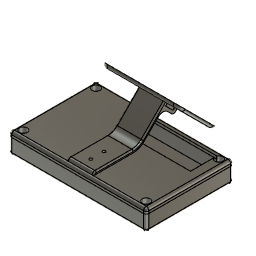
LCD 2004 (Autodesk Fusion 360 design; units mm, degrees)
Autodesk Fusion 360 part; units mm, degrees
sketch "base" plane through (0, 0, 0) normal (0, 0, 1) x (1, 0, 0)
  line L0 (0, 0) -> (104, 0)
  line L1 (104, 0) -> (104, 66)
  line L2 (104, 66) -> (0, 66)
  line L3 (0, 66) -> (0, 0)
  line L4 (2, 53) -> (102, 53)
  line L5 (102, 53) -> (102, 13)
  line L6 (102, 13) -> (2, 13)
  line L7 (2, 13) -> (2, 53)
  line L8 (2, 53) -> (102, 53)
  line L9 (102, 53) -> (102, 64)
  line L10 (102, 64) -> (2, 64)
  line L11 (2, 64) -> (2, 53)
  line L12 (2, 13) -> (102, 13)
  line L13 (102, 13) -> (102, 2)
  line L14 (102, 2) -> (2, 2)
  line L15 (2, 2) -> (2, 13)
  line L16 (2, 53) -> (3, 53)
  line L17 (3, 53) -> (3, 13)
  line L18 (3, 13) -> (2, 13)
  line L19 (2, 13) -> (2, 53)
  line L20 (102, 53) -> (101, 53)
  line L21 (101, 53) -> (101, 13)
  line L22 (101, 13) -> (102, 13)
  line L23 (102, 13) -> (102, 53)
  dimension "d1" = 104
  dimension "d2" = 66
  dimension "d3" = 100
  dimension "d4" = 40
  dimension "d6" = 2
  dimension "d8" = 11
  dimension "d10" = 11
  dimension "d41" = 2
  dimension "d46" = 1
  dimension "d47" = 1
  constraint horizontal L0
  constraint vertical L1
  constraint horizontal L2
  constraint vertical L3
  constraint coincident L0.start L3.end
  constraint horizontal L4
  constraint vertical L5
  constraint horizontal L6
  constraint vertical L7
  constraint horizontal L8
  constraint vertical L9
  constraint horizontal L10
  constraint vertical L11
  constraint horizontal L12
  constraint vertical L13
  constraint horizontal L14
  constraint vertical L15
  constraint coincident L5.end L13
  constraint coincident L4.end L9
  constraint horizontal L16
  constraint vertical L17
  constraint horizontal L18
  constraint vertical L19
  constraint horizontal L20
  constraint vertical L21
  constraint horizontal L22
  constraint vertical L23
  measures "d1" distance of L0.start L0.end
  measures "d2" distance of L0.start L2.end
  measures "d3" distance of L4.start L4.end
  measures "d4" distance of L4.start L6.end
  measures "d6" distance of L3 L7
  measures "d8" distance of L4.start L10.end
  measures "d10" distance of L6.end L14.end
  measures "d41" distance of L2 L10
  measures "d46" distance of L4.start L16.end
  measures "d47" distance of L4.end L20.end
extrude "Extrude1" add sketch "base" along normal blind 2 contours L4 L8 L9 L10 L11 L16 L20 | L4 L6 L7 L8 L12 L16 L17 L18 L19 | L6 L12 L13 L14 L15 L18 L22 | L4 L5 L6 L8 L12 L20 L21 L22 L23 makes body 1
extrude "Extrude2" add sketch "base" along normal blind 12 bodies 1
fillet "Fillet1" radius 2 4 edges at (0, 0, 6) (0, 66, 6) (104, 66, 6) (104, 0, 6) on bodies 1
fillet "Fillet2" radius 2 8 edges at (104, 33, 0) (103.4142, 65.4142, 0) (52, 66, 0) (0.5858, 65.4142, 0) (0, 33, 0) (0.5858, 0.5858, 0) (52, 0, 0) (103.4142, 0.5858, 0) on bodies 1
sketch "stands " plane through (0, 0, 2) normal (0, 0, 1) x (-1, 0, 0)
  line L0 (-2, -2) -> (-102, -2)
  line L1 (-102, -2) -> (-102, -64)
  line L2 (-101, -13) -> (-3, -13)
  line L3 (-2, -64) -> (-2, -2)
  line L4 (-2, -64) -> (-11, -64)
  line L5 (-11, -64) -> (-11, -55)
  line L6 (-11, -55) -> (-2, -55)
  line L7 (-2, -55) -> (-2, -64)
  line L8 (-102, -64) -> (-93, -64)
  line L9 (-93, -64) -> (-93, -55)
  line L10 (-93, -55) -> (-102, -55)
  line L11 (-102, -55) -> (-102, -64)
  line L12 (-102, -2) -> (-93, -2)
  line L13 (-93, -2) -> (-93, -11)
  line L14 (-93, -11) -> (-102, -11)
  line L15 (-102, -11) -> (-102, -2)
  line L16 (-2, -2) -> (-11, -2)
  line L17 (-11, -2) -> (-11, -11)
  line L18 (-11, -11) -> (-2, -11)
  line L19 (-2, -11) -> (-2, -2)
  circle A0 centre (-5.4, -60.6) radius 2.2
  circle A1 centre (-98.6, -60.6) radius 2.2
  circle A2 centre (-98.6, -5.4) radius 2.2
  circle A3 centre (-5.4, -5.4) radius 2.2
  line L20 (-3, -13) -> (-3, -53)
  line L21 (-3, -53) -> (-101, -53)
  line L22 (-101, -53) -> (-101, -13)
  line L23 (-102, -64) -> (-2, -64)
  point P0 (-2, -64)
  point P1 (-102, -64)
  dimension "d19" = 9
  dimension "d20" = 9
  dimension "d21" = 9
  dimension "d22" = 9
  dimension "d23" = 9
  dimension "d24" = 9
  dimension "d25" = 9
  dimension "d26" = 9
  dimension "d29" = 4.4
  dimension "d30" = 4.4
  dimension "d31" = 4.4
  dimension "d32" = 4.4
  dimension "d33" = 3.4
  dimension "d34" = 3.4
  dimension "d35" = 3.4
  dimension "d36" = 3.4
  dimension "d37" = 3.4
  dimension "d38" = 3.4
  dimension "d39" = 3.4
  dimension "d40" = 3.4
  constraint horizontal L4
  constraint vertical L5
  constraint horizontal L6
  constraint vertical L7
  constraint horizontal L8
  constraint vertical L9
  constraint horizontal L10
  constraint vertical L11
  constraint horizontal L12
  constraint vertical L13
  constraint horizontal L14
  constraint vertical L15
  constraint coincident L0.end L1.start
  constraint horizontal L16
  constraint vertical L17
  constraint horizontal L18
  constraint vertical L19
  constraint coincident L0.start L3.end
  constraint coincident L4 P0
  constraint coincident L7 P0
  constraint coincident L8 P1
  constraint coincident L11 P1
  measures "d19" distance of P0 L4.end
  measures "d20" distance of P0 L6.end
  measures "d21" distance of P1 L8.end
  measures "d22" distance of P1 L10.end
  measures "d23" distance of L0.end L12.end
  measures "d24" distance of L0.end L14.end
  measures "d25" distance of L0.start L16.end
  measures "d26" distance of L0.start L18.end
  measures "d29" diameter of A0
  measures "d30" diameter of A1
  measures "d31" diameter of A2
  measures "d32" diameter of A3
  measures "d33" distance of L19 A3.centre
  measures "d34" distance of L16 A3.centre
  measures "d35" distance of L15 A2.centre
  measures "d36" distance of L12 A2.centre
  measures "d37" distance of L11 A1.centre
  measures "d38" distance of L8 A1.centre
  measures "d39" distance of L7 A0.centre
  measures "d40" distance of L4 A0.centre
extrude "Extrude3" add sketch "stands " along normal blind 6 contours L0 L3 L16 L17 L18 L19 | L0 L1 L12 L13 L14 L15 | L3 L4 L5 L6 L7 L23 | L1 L8 L9 L10 L11 L23 bodies 1
extrude "Extrude21" cut 4 faces at (98.9667, 6.2537, 2) (6.0465, 4.7174, 2) (4.8624, 59.6689, 2) (98.9667, 61.4537, 2) along direction (0, 0, -1) blind 1 on bodies 1 bodies 1
fillet "Fillet3" radius 2 8 edges at (11, 64, 5) (2, 55, 5) (2, 11, 5) (11, 2, 5) (93, 2, 5) (102, 11, 5) (102, 55, 5) (93, 64, 5) on bodies 1
fillet "Fillet4" radius 3.5 4 edges at (93, 55, 5) (93, 11, 5) (11, 11, 5) (11, 55, 5) on bodies 1
fillet "Fillet5" radius 1 4 edges at (3, 53, 1) (101, 53, 1) (101, 13, 1) (3, 13, 1) on bodies 1
chamfer "Chamfer1" distance 0.5 angle 45 4 edges at (100.6511, 4.6044, 8) (7.4511, 4.6044, 8) (7.4511, 59.8044, 8) (100.6511, 59.8044, 8) on bodies 1
sketch "Sketch3" plane through (0, 0, 0) normal (0, 0, 1) x (1, 0, 0)
  line L0 (0, 0) -> (-104, 0)
  line L1 (-104, 0) -> (-104, 66)
  line L2 (-104, 66) -> (0, 66)
  line L3 (0, 66) -> (0, 0)
  line L4 (-95.8, 61.8) -> (-43.8, 61.8)
  line L5 (-43.8, 61.8) -> (-43.8, 41.8)
  line L6 (-43.8, 41.8) -> (-95.8, 41.8)
  line L7 (-95.8, 41.8) -> (-95.8, 61.8)
  line L8 (-101.8, 63.8) -> (-2.2, 63.8)
  line L9 (-2.2, 63.8) -> (-2.2, 2.2)
  line L10 (-2.2, 2.2) -> (-101.8, 2.2)
  line L11 (-101.8, 2.2) -> (-101.8, 63.8)
  dimension "d51" = 104
  dimension "d52" = 66
  dimension "d69" = 52
  dimension "d70" = 20
  dimension "d71" = 4.2
  dimension "d72" = 8.2
  dimension "d73" = 99.6
  dimension "d74" = 61.6
  dimension "d75" = 2.2
  dimension "d76" = 2.2
  constraint horizontal L0
  constraint vertical L1
  constraint horizontal L2
  constraint vertical L3
  constraint coincident L0.start L3.end
  constraint horizontal L4
  constraint vertical L5
  constraint horizontal L6
  constraint vertical L7
  constraint horizontal L8
  constraint vertical L9
  constraint horizontal L10
  constraint vertical L11
  measures "d51" distance of L0.start L0.end
  measures "d52" distance of L0.start L2.end
  measures "d69" distance of L4.start L4.end
  measures "d70" distance of L4.start L6.end
  measures "d71" distance of L2 L4
  measures "d72" distance of L1 L7
  measures "d73" distance of L8.start L8.end
  measures "d74" distance of L8.start L10.end
  measures "d75" distance of L2 L8
  measures "d76" distance of L1 L11
extrude "Extrude4" add sketch "Sketch3" along normal blind 2 separate body contours L8 L9 L10 L11 makes body 2
sketch "Sketch4" plane through (0, 0, 2) normal (0, 0, 1) x (-1, 0, 0)
  line L0 (2.2, -2.2) -> (101.8, -2.2)
  line L1 (101.8, -2.2) -> (101.8, -63.8)
  line L2 (101.8, -63.8) -> (2.2, -63.8)
  line L3 (2.2, -63.8) -> (2.2, -2.2)
  line L4 (101.8, -63.8) -> (95.8, -63.8)
  line L5 (95.8, -63.8) -> (95.8, -55.8)
  line L6 (95.8, -55.8) -> (101.8, -55.8)
  line L7 (101.8, -55.8) -> (101.8, -63.8)
  line L8 (2.2, -63.8) -> (10.2, -63.8)
  line L9 (10.2, -63.8) -> (10.2, -55.8)
  line L10 (10.2, -55.8) -> (2.2, -55.8)
  line L11 (2.2, -55.8) -> (2.2, -63.8)
  line L12 (2.2, -2.2) -> (10.2, -2.2)
  line L13 (10.2, -2.2) -> (10.2, -10.2)
  line L14 (10.2, -10.2) -> (2.2, -10.2)
  line L15 (2.2, -10.2) -> (2.2, -2.2)
  line L16 (101.8, -2.2) -> (93.8, -2.2)
  line L17 (93.8, -2.2) -> (93.8, -10.2)
  line L18 (93.8, -10.2) -> (101.8, -10.2)
  line L19 (101.8, -10.2) -> (101.8, -2.2)
  line L20 (43.8, -41.8) -> (95.8, -41.8)
  line L21 (95.8, -41.8) -> (95.8, -61.8)
  line L22 (95.8, -61.8) -> (43.8, -61.8)
  line L23 (43.8, -61.8) -> (43.8, -41.8)
  line L24 (101.8, -2.2) -> (2.2, -2.2)
  line L25 (2.2, -2.2) -> (2.2, -63.8)
  line L26 (2.2, -63.8) -> (101.8, -63.8)
  line L27 (101.8, -63.8) -> (101.8, -2.2)
  dimension "d55" = 99.6
  dimension "d56" = 61.6
  dimension "d59" = 6
  dimension "d60" = 8
  dimension "d61" = 8
  dimension "d62" = 8
  dimension "d63" = 8
  dimension "d64" = 8
  dimension "d65" = 8
  dimension "d66" = 8
  constraint horizontal L0
  constraint vertical L1
  constraint horizontal L2
  constraint vertical L3
  constraint horizontal L4
  constraint vertical L5
  constraint horizontal L6
  constraint vertical L7
  constraint horizontal L8
  constraint vertical L9
  constraint horizontal L10
  constraint vertical L11
  constraint horizontal L12
  constraint vertical L13
  constraint horizontal L14
  constraint vertical L15
  constraint horizontal L16
  constraint vertical L17
  constraint horizontal L18
  constraint vertical L19
  constraint coincident L2 L1.end
  constraint coincident L7 L1.end
  measures "d55" distance of L1.end L2.end
  measures "d56" distance of L0.end L1.end
  measures "d59" distance of L1.end L4.end
  measures "d60" distance of L1.end L6.end
  measures "d61" distance of L2.end L8.end
  measures "d62" distance of L2.end L10.end
  measures "d63" distance of L0.start L12.end
  measures "d64" distance of L0.start L14.end
  measures "d65" distance of L0.end L16.end
  measures "d66" distance of L0.end L18.end
extrude "Extrude5" add sketch "Sketch4" along normal blind 4 contours L0 L3 L12 L13 L14 L15 L24 L25 | L0 L1 L16 L17 L18 L19 L24 L27 | L2 L3 L8 L9 L10 L11 L25 L26 | L1 L2 L4 L5 L6 L7 L21 L26 L27 bodies 2
extrude "Extrude6" add sketch "Sketch3" along normal blind 3.8 contours L0 L1 L2 L3 bodies 2
sketch "Sketch9" plane through (0, 0, 0) normal (0, 0, -1) x (1, 0, 0)
  line L0 (-104, 0) -> (-104, -66)
  line L1 (-104, -66) -> (0, -66)
  line L2 (0, -66) -> (0, 0)
  line L3 (0, 0) -> (-104, 0)
  line L4 (-95.8, -41.8) -> (-43.8, -41.8)
  line L5 (-43.8, -41.8) -> (-43.8, -61.8)
  line L6 (-43.8, -61.8) -> (-95.8, -61.8)
  line L7 (-95.8, -61.8) -> (-95.8, -41.8)
  line L8 (-43.8, -41.8) -> (-75.8, -41.8)
  line L9 (-75.8, -41.8) -> (-75.8, -39.8)
  line L10 (-75.8, -39.8) -> (-43.8, -39.8)
  line L11 (-43.8, -39.8) -> (-43.8, -41.8)
  line L12 (-43.8, -61.8) -> (-75.8, -61.8)
  line L13 (-75.8, -61.8) -> (-75.8, -63.8)
  line L14 (-75.8, -63.8) -> (-43.8, -63.8)
  line L15 (-43.8, -63.8) -> (-43.8, -61.8)
  line L16 (-43.8, -63.8) -> (-41.8, -63.8)
  line L17 (-41.8, -63.8) -> (-41.8, -39.8)
  line L18 (-41.8, -39.8) -> (-43.8, -39.8)
  line L19 (-43.8, -39.8) -> (-43.8, -63.8)
  line L20 (-95.8, -57.8) -> (-97.8, -57.8)
  line L21 (-97.8, -57.8) -> (-97.8, -39.8)
  line L22 (-97.8, -39.8) -> (-95.8, -39.8)
  line L23 (-95.8, -39.8) -> (-95.8, -57.8)
  dimension "d147" = 32
  dimension "d148" = 2
  dimension "d149" = 32
  dimension "d150" = 2
  dimension "d151" = 2
  dimension "d152" = 24
  dimension "d153" = 2
  dimension "d154" = 18
  constraint horizontal L8
  constraint vertical L9
  constraint horizontal L10
  constraint vertical L11
  constraint coincident L4.end L5.start
  constraint horizontal L12
  constraint vertical L13
  constraint horizontal L14
  constraint vertical L15
  constraint coincident L5.end L6.start
  constraint horizontal L16
  constraint vertical L17
  constraint horizontal L18
  constraint vertical L19
  constraint horizontal L20
  constraint vertical L21
  constraint horizontal L22
  constraint vertical L23
  constraint coincident L4.start L23
  constraint coincident L9.end L22
  measures "d147" distance of L4.end L8.end
  measures "d148" distance of L4.end L10.end
  measures "d149" distance of L5.end L12.end
  measures "d150" distance of L5.end L14.end
  measures "d151" distance of L14.end L16.end
  measures "d152" distance of L14.end L10.end
  measures "d153" distance of L20.start L20.end
  measures "d154" distance of L20.start L22.end
fillet "Fillet6" radius 2 4 edges at (-104, 66, 1.9) (0, 66, 1.9) (0, 0, 1.9) (-104, 0, 1.9) on bodies 2
fillet "Fillet7" radius 2 4 edges at (-101.8, 2.2, 4.9) (-101.8, 63.8, 4.9) (-2.2, 63.8, 4.9) (-2.2, 2.2, 4.9) on bodies 2
sketch "Sketch7" plane through (0, 0, 0) normal (0, 0, -1) x (1, 0, 0)
  arc A0 (-102, 0) -> (-104, -2) centre (-102, -2) ccw
  line L0 (-104, -2) -> (-104, -64)
  arc A1 (-104, -64) -> (-102, -66) centre (-102, -64) ccw
  line L1 (-102, -66) -> (-2, -66)
  arc A2 (-2, -66) -> (0, -64) centre (-2, -64) ccw
  line L2 (0, -64) -> (0, -2)
  arc A3 (0, -2) -> (-2, 0) centre (-2, -2) ccw
  line L3 (-2, 0) -> (-102, 0)
  line L4 (-95.8, -41.8) -> (-43.8, -41.8)
  line L5 (-43.8, -41.8) -> (-43.8, -61.8)
  line L6 (-43.8, -61.8) -> (-95.8, -61.8)
  line L7 (-95.8, -61.8) -> (-95.8, -41.8)
  circle A4 centre (-98.6, -5.4) radius 1.7
  circle A5 centre (-98.6, -5.4) radius 3
  circle A6 centre (-5.4, -5.4) radius 1.7
  circle A7 centre (-5.4, -5.4) radius 3
  circle A8 centre (-5.4, -60.6) radius 1.7
  circle A9 centre (-5.4, -60.6) radius 3
  circle A10 centre (-98.6, -60.6) radius 1.7
  circle A11 centre (-98.6, -60.6) radius 3
  line L8 (-52, -66) -> (-52, 0) construction
  circle A12 centre (-52, -10) radius 1.1
  circle A13 centre (-52, -20) radius 1.1
  dimension "d117" = 3.4
  dimension "d118" = 6
  dimension "d119" = 3.4
  dimension "d120" = 6
  dimension "d121" = 3.4
  dimension "d122" = 6
  dimension "d123" = 3.4
  dimension "d124" = 6
  dimension "d125" = 5.4
  dimension "d126" = 5.4
  dimension "d127" = 5.4
  dimension "d128" = 5.4
  dimension "d129" = 5.4
  dimension "d130" = 5.4
  dimension "d131" = 5.4
  dimension "d132" = 5.4
  dimension "d239" = 2.2
  dimension "d240" = 2.2
  dimension "d241" = 10
  dimension "d242" = 10
  constraint concentric A4 A5
  constraint concentric A6 A7
  constraint concentric A8 A9
  constraint concentric A10 A11
  constraint midpoint L1 L8.start
  constraint midpoint L3 L8.end
  constraint coincident L8 A12.centre
  constraint coincident L8 A13.centre
  measures "d117" diameter of A4
  measures "d118" diameter of A5
  measures "d119" diameter of A6
  measures "d120" diameter of A7
  measures "d121" diameter of A8
  measures "d122" diameter of A9
  measures "d123" diameter of A10
  measures "d124" diameter of A11
  measures "d125" distance of L0 A10.centre
  measures "d126" distance of L1 A10.centre
  measures "d127" distance of L1 A8.centre
  measures "d128" distance of L2 A8.centre
  measures "d129" distance of L2 A6.centre
  measures "d130" distance of L3 A6.centre
  measures "d131" distance of L0 A4.centre
  measures "d132" distance of L3 A4.centre
  measures "d239" diameter of A12
  measures "d240" diameter of A13
  measures "d241" distance of L3 A12.centre
  measures "d242" distance of A12.centre A13.centre
extrude "Extrude7" cut sketch "Sketch7" against normal blind 6 contours A4 | A6 | A8 | A10 bodies 1 2
extrude "Extrude8" cut sketch "Sketch7" against normal blind 4 contours L7 A11 | L7 A11 | A5 | A7 | A9 bodies 2
fillet "Fillet8" radius 2 12 edges at (-10.2, 55.8, 4) (-2.2, 55.8, 4.9) (-10.2, 63.8, 4.9) (-10.2, 2.2, 4.9) (-10.2, 10.2, 4) (-2.2, 10.2, 4.9) (-101.8, 10.2, 4.9) (-93.8, 10.2, 4) (-93.8, 2.2, 4.9) (-101.8, 55.8, 4.9) (-95.8, 55.8, 4) (-95.8, 63.8, 4.9) on bodies 2
fillet "Fillet9" radius 2 8 edges at (-103.4142, 0.5858, 0) (-104, 33, 0) (-103.4142, 65.4142, 0) (-52, 66, 0) (-0.5858, 65.4142, 0) (0, 33, 0) (-0.5858, 0.5858, 0) (-52, 0, 0) on bodies 2
sketch "Sketch11" plane through (0, 0, 0) normal (0, 0, 1) x (1, 0, 0)
  line L0 (0, -45) -> (2, -45)
  line L1 (2, -45) -> (2, -80)
  line L2 (2, -80) -> (0, -80)
  line L3 (0, -80) -> (0, -45)
  line L4 (2, -45) -> (14.7279, -45) construction
  line L5 (0, -45) -> (17.6777, -27.3223)
  line L6 (0, -45) -> (25, -45) construction
  line L7 (17.6777, -27.3223) -> (19.0919, -28.7365)
  line L8 (17.6777, -27.3223) -> (19.6777, -27.3223) construction
  line L9 (19.0919, -28.7365) -> (2, -45.8284)
  line L10 (17.6777, -27.3223) -> (16.6894, -26.334)
  line L11 (16.6894, -26.334) -> (9.6183, -19.263)
  line L12 (9.6183, -19.263) -> (12.4467, -16.4345)
  line L13 (9.6183, -19.263) -> (11.6183, -19.263) construction
  line L14 (19.0919, -28.7365) -> (21.9203, -25.9081)
  line L15 (19.0919, -28.7365) -> (21.0919, -28.7365) construction
  line L16 (12.4467, -16.4345) -> (21.9203, -25.9081)
  dimension "d165" = 2
  dimension "d166" = 35
  dimension "d169" = 45
  dimension "d170" = 25
  dimension "d171" = 45
  dimension "d172" = 2
  dimension "d173" = 10
  dimension "d174" = 45
  dimension "d176" = 45
  dimension "d190" = 4
  constraint horizontal L0
  constraint vertical L1
  constraint horizontal L2
  constraint vertical L3
  constraint horizontal L4
  constraint horizontal L6
  constraint horizontal L8
  constraint coincident L1 L9.end
  constraint perpendicular L7 L9
  constraint perpendicular L5 L11
  constraint horizontal L13
  constraint horizontal L15
  constraint perpendicular L14 L16
  measures "d165" distance of L0.start L0.end
  measures "d166" distance of L0.start L2.end
  measures "d169" angle of L5 L6
  measures "d170" distance of L0.start L5.end
  measures "d171" angle of L7 L8
  measures "d172" distance of L5.end L7.end
  measures "d173" distance of L10.end L11.end
  measures "d174" angle of L12 L13
  measures "d176" angle of L14 L15
  measures "d190" distance of L11.end L12.end
extrude "Extrude12" add sketch "Sketch11" along normal blind 20 separate body makes body 3
fillet "Fillet10" radius 10 1 edges at (2, -45.8284, 10) on bodies 3
fillet "Fillet11" radius 12 1 edges at (0, -45, 10) on bodies 3
fillet "Fillet12" radius 5 1 edges at (17.6777, -27.3223, 10) on bodies 3
sketch "Sketch13" plane through (-1.9939, -1.9939, 0) normal (0.707107, 0.707107, 0) x (-0.707107, 0.707107, 0)
  line L0 (-33.8198, 0) -> (-20.4221, 0)
  line L1 (-20.4221, 0) -> (-20.4221, 20)
  line L2 (-20.4221, 20) -> (-33.8198, 20)
  line L3 (-33.8198, 20) -> (-33.8198, 0)
  line L4 (-27.121, 20) -> (-27.121, 0) construction
  circle A0 centre (-27.121, 15) radius 2.5
  circle A1 centre (-27.121, 5) radius 2.5
  circle A2 centre (-27.121, 5) radius 1.1
  circle A3 centre (-27.121, 15) radius 1.1
  line L5 (-30.9218, 20) -> (-22.9221, 20)
  line L6 (-22.9221, 20) -> (-22.9221, 0)
  line L7 (-22.9221, 0) -> (-30.9218, 0)
  line L8 (-30.9218, 0) -> (-30.9218, 20)
  dimension "d191" = 5
  dimension "d192" = 5
  dimension "d193" = 2.2
  dimension "d194" = 2.2
  dimension "d195" = 5
  dimension "d196" = 5
  dimension "d201" = 7.9997
  dimension "d202" = 2.5
  constraint midpoint L2 L4.start
  constraint midpoint L0 L4.end
  constraint coincident L4 A0.centre
  constraint coincident L4 A1.centre
  constraint concentric A1 A2
  constraint concentric A0 A3
  constraint horizontal L5
  constraint vertical L6
  constraint horizontal L7
  constraint vertical L8
  constraint coincident L0 L6.end
  constraint coincident L2 L5.start
  measures "d191" diameter of A0
  measures "d192" diameter of A1
  measures "d193" diameter of A2
  measures "d194" diameter of A3
  measures "d195" distance of L2 A0.centre
  measures "d196" distance of L0 A1.centre
  measures "d201" distance of L6 L8
  measures "d202" distance of L1 L6
extrude "Extrude13" cut sketch "Sketch13" against normal blind 5 contours A0 | A1 | A2 | A3 bodies 3
extrude "Extrude14" add sketch "Sketch13" against normal blind 4 contours A0 | A1 bodies 3
extrude "Extrude15" cut sketch "Sketch13" against normal blind 2 contours L0 L2 L5 L6 L7 L8 | A0 | A1 | A2 | A3 bodies 3
fillet "Fillet13" radius 2 1 edges at (2, -80, 10) on bodies 3
fillet "Fillet14" radius 2 1 edges at (9.6183, -19.263, 10) on bodies 3
fillet "Fillet15" radius 1 4 edges at (1.4142, -79.4142, 20) (2, -63.9853, 20) (2.7612, -46.1437, 20) (13.4246, -34.4038, 20) on bodies 3
fillet "Fillet16" radius 1 4 edges at (13.4246, -34.4038, 0) (2.7612, -46.1437, 0) (2, -63.9853, 0) (1.4142, -79.4142, 0) on bodies 3
sketch "Sketch14" plane through (0, 0, 0) normal (0, 0, 1) x (1, 0, 0)
  line L0 (-85, -25) -> (-25, -25)
  line L1 (-25, -25) -> (-25, -65)
  line L2 (-25, -65) -> (-85, -65)
  line L3 (-85, -65) -> (-85, -25)
  dimension "d213" = 60
  dimension "d214" = 40
  constraint horizontal L0
  constraint vertical L1
  constraint horizontal L2
  constraint vertical L3
  measures "d213" distance of L0.start L0.end
  measures "d214" distance of L0.start L2.end
extrude "Extrude16" add sketch "Sketch14" along normal blind 2 separate body makes body 4
sketch "Sketch15" plane through (0, 0, 2) normal (0, 0, 1) x (-1, 0, 0)
  line L0 (85, 65) -> (25, 65)
  line L1 (25, 65) -> (25, 25)
  line L2 (25, 25) -> (85, 25)
  line L3 (85, 25) -> (85, 65)
  line L4 (65, 41.2) -> (45, 41.2)
  line L5 (45, 41.2) -> (45, 48.8)
  line L6 (45, 48.8) -> (65, 48.8)
  line L7 (65, 48.8) -> (65, 41.2)
  line L8 (65, 45) -> (45, 45) construction
  circle A0 centre (60, 45) radius 1.1
  circle A1 centre (60, 45) radius 2
  circle A2 centre (50, 45) radius 1.1
  circle A3 centre (50, 45) radius 2
  dimension "d217" = 20
  dimension "d218" = 7.6
  dimension "d219" = 20
  dimension "d220" = 16.2
  dimension "d221" = 4
  dimension "d222" = 2.2
  dimension "d223" = 2.2
  dimension "d224" = 4
  dimension "d225" = 5
  dimension "d226" = 5
  constraint horizontal L4
  constraint vertical L5
  constraint horizontal L6
  constraint vertical L7
  constraint midpoint L7 L8.start
  constraint midpoint L5 L8.end
  constraint coincident L8 A0.centre
  constraint concentric A0 A1
  constraint coincident L8 A2.centre
  constraint concentric A2 A3
  measures "d217" distance of L4.start L4.end
  measures "d218" distance of L4.start L6.end
  measures "d219" distance of L3 L7
  measures "d220" distance of L0 L6
  measures "d221" diameter of A1
  measures "d222" diameter of A0
  measures "d223" diameter of A2
  measures "d224" diameter of A3
  measures "d225" distance of L5 A2.centre
  measures "d226" distance of L7 A0.centre
extrude "Extrude18" cut sketch "Sketch15" against normal blind 2 contours A0 | A1 | A2 | A3 bodies 4
extrude "Extrude17" add sketch "Sketch15" along normal blind 1.8 contours L4 L5 L6 L7 | A1 | A3 bodies 4
fillet "Fillet17" radius 5 4 edges at (-85, -65, 1) (-85, -25, 1) (-25, -65, 1) (-25, -25, 1) on bodies 4
fillet "Fillet18" radius 2 8 edges at (-26.4645, -63.5355, 2) (-25, -45, 2) (-26.4645, -26.4645, 2) (-55, -25, 2) (-83.5355, -26.4645, 2) (-85, -45, 2) (-83.5355, -63.5355, 2) (-55, -65, 2) on bodies 4
extrude "Extrude19" cut sketch "Sketch7" against normal blind 4 contours A12 | A13 bodies 2
sketch "Sketch16" plane through (0, 0, 0) normal (-1, 0, 0) x (0, -1, 0)
  arc A0 (79, 0) -> (80, 1) centre (79, 1) ccw
  line L0 (80, 1) -> (80, 19)
  arc A1 (80, 19) -> (79, 20) centre (79, 19) ccw
  line L1 (79, 20) -> (49.9706, 20)
  line L2 (49.9706, 20) -> (49.9706, 0)
  line L3 (49.9706, 0) -> (79, 0)
  line L4 (49.9706, 10) -> (80, 10) construction
  circle A2 centre (72, 10) radius 1.1
  circle A3 centre (62, 10) radius 1.1
  dimension "d245" = 2.2
  dimension "d246" = 2.2
  dimension "d247" = 8
  dimension "d248" = 10
  constraint midpoint L2 L4.start
  constraint midpoint L0 L4.end
  constraint coincident L4 A2.centre
  constraint coincident L4 A3.centre
  measures "d245" diameter of A2
  measures "d246" diameter of A3
  measures "d247" distance of L0 A2.centre
  measures "d248" distance of A2.centre A3.centre
extrude "Extrude20" cut sketch "Sketch16" against normal blind 3 contours A2 | A3 bodies 3
copy_body "Body->Comp3" bodies 2 removing the originals makes body 5 in component "back lid"
copy_body "Body->Comp4" bodies 1 removing the originals makes body 6 in component "base"
extrude "Extrude1'" cut sketch "stands " against normal blind 1 contours A0 | A1 | A2 | A3 bodies 6 in component "base"
copy_body "Body->Comp5" bodies 3 removing the originals makes body 7 in component "mount"
copy_body "Body->Comp6" bodies 4 removing the originals makes body 8 in component "mount plate"
component "back lid" placed x (-1, 0, 0) y (0, 1, 0) z (0, 0, -1) at (0, 0, 15.8)
component "base" placed x (1, 0, 0) y (0, 1, 0) z (0, 0, 1) at (0, 0, 0)
component "mount" placed x (0, 0, 1) y (0, 1, 0) z (-1, 0, 0) at (62, 82, 15.8)
component "mount plate" placed x (1, 0, 0) y (0, -0.707107, 0.707107) z (0, -0.707107, -0.707107) at (107, 30.4224, 65.9354)
named bodies: "base", "back lid", "mount", "mount plate"
